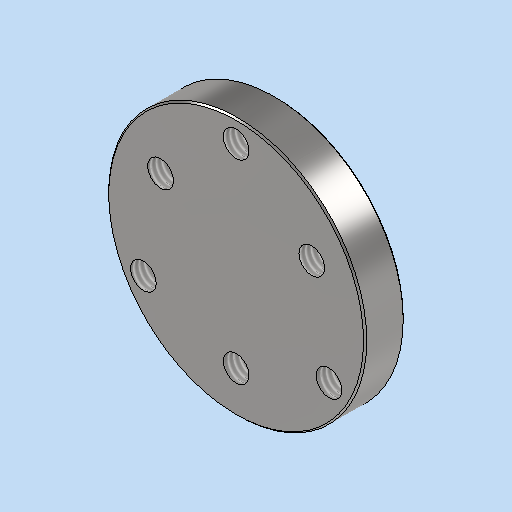
# Autodesk Inventor part: flange-adapter
Saved by Autodesk Inventor 2026 (Build 300175050, 175E)
## iProperties
Created: 2025-06-19
Part Number: flange-adapter
Material: Stainless Steel
Document SubType Name: Modeling
Designer: kuzmin
Density: 8 g/cm^3
Appearance: Semi-Polished
Author: kuzmin
Autodesk Inventor part; units mm, degrees
ref_plane "YZ Plane" through (0, 0, 0) normal (1, 0, 0) x (0, 1, 0)
ref_plane "XZ Plane" through (0, 0, 0) normal (0, 1, 0) x (-1, 0, 0)
ref_plane "XY Plane" through (0, 0, 0) normal (0, 0, 1) x (1, 0, 0)
sketch "Sketch1" plane through (0, 0, 0) normal (0, 0, 1) x (1, 0, 0)
  circle A0 centre (0, 0) radius 16.25
  circle A1 centre (0, 0) radius 13.5 construction
  circle A2 centre (0, 0) radius 11 construction
  line L0 (0, 13.5) -> (0, 0) construction
  line L1 (0, 0) -> (9.5263, 5.5) construction
  dimension "d2" = 22
  dimension "d0" = 32.5
  dimension "d1" = 27
  dimension "d3" = 60
  constraints: 4 end point, 3 coincident, 2 centre point, 2 point on circle, 1 vertical, 3 other
  measures "d0" diameter of A0
  measures "d1" diameter of A1
  measures "d3" angle of L0 L1
extrude "Extrusion1" add sketch "Sketch1" along normal blind 5
hole "Hole1" at (0, 13.5, 0) at (9.5263, 5.5, 0) direction (0, 0, 1) diameter 3.242 depth 5 thread size "M4x0.7" class "6H" standard "ANSI Metric M Profile"
pattern_circular "Circular Pattern1" count 3 over 360 about axis through (0, 0, 0) along (0, 0, 1) of "Hole1"
chamfer "Chamfer1" distance 0.2 angle 45 2 edges at (-16.25, 0, 5) (-16.25, 0, 0)
equation "\"d2\" = holesid"
equation "\"holesid\" = 22"
body "Solid1"
